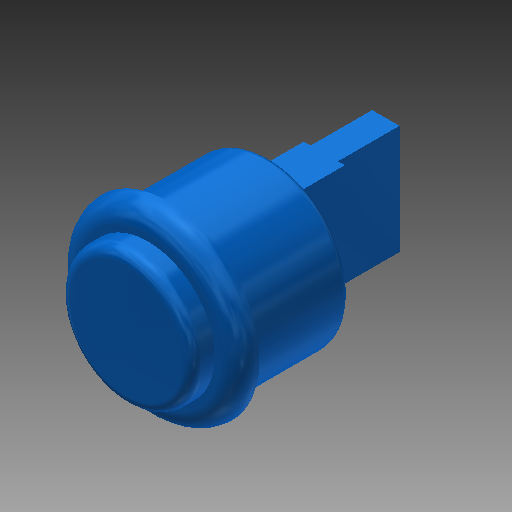
# Autodesk Inventor part: OBSF-24_button
Saved by Autodesk Inventor 2019 (Build 230136000, 136)
## iProperties
Created: 2013-02-11
Part Number: OBSF-24_button
Material: Nylon 6
Document SubType Name: Modeling
Designer: mstine
Density: 1 g/cm^3
Appearance: Nylon 6
Author: mstine
Autodesk Inventor part; units mm, degrees
ref_plane "YZ Plane" through (0, 0, 0) normal (1, 0, 0) x (0, 1, 0)
ref_plane "XZ Plane" through (0, 0, 0) normal (0, 1, 0) x (-1, 0, 0)
ref_plane "XY Plane" through (0, 0, 0) normal (0, 0, 1) x (1, 0, 0)
sketch "Sketch1" plane through (0, 0, 0) normal (0, 0, 1) x (1, 0, 0)
  circle A0 centre (0, 0) radius 11.75
  dimension "d0" = 23.5
  constraints: 1 centre point, 1 coincident
  measures "d0" diameter of A0
extrude "Extrusion1" add sketch "Sketch1" against normal blind 15
sketch "Sketch2" plane through (0, 0, 0) normal (0, 0, 1) x (1, 0, 0)
  circle A0 centre (0, 0) radius 11.75 projected
  circle A1 centre (0, 0) radius 13.5
  dimension "d3" = 27
  constraints: 1 centre point, 1 coincident
  measures "d3" diameter of A1
extrude "Extrusion2" add sketch "Sketch2" along normal blind 2.8 contours A0 | A1
sketch "Sketch3" plane through (0, 0, 2.8) normal (0, 0, 1) x (1, 0, 0)
  circle A0 centre (0, 0) radius 13.5 projected
  circle A1 centre (0, 0) radius 9.75
  dimension "d8" = 19.5
  constraints: 1 centre point, 1 coincident
  measures "d8" diameter of A1
extrude "Extrusion3" add sketch "Sketch3" along normal blind 3.2 contours A1
fillet "Fillet1" radius 1.5 1 edges at (-9.75, 0, 6)
fillet "Fillet2" radius 2.95 1 edges at (-13.5, 0, 2.8)
fillet "Fillet3" radius 1 1 edges at (-11.75, 0, -15)
sketch "Sketch4" plane through (0, 0, -15) normal (0, 0, -1) x (-1, 0, 0)
  circle A0 centre (0, 0) radius 10.75 projected
  line L0 (-3, 8) -> (3, 8)
  line L1 (3, 8) -> (3, -8)
  line L2 (3, -8) -> (-3, -8)
  line L3 (-3, -8) -> (-3, 8)
  point P0 (3, 0)
  point P1 (0, 8)
  dimension "d14" = 6
  dimension "d16" = 16
  constraints: 8 end point, 2 midpoint, 2 parallel, 1 horizontal, 1 horizontal alignment, 1 perpendicular, 1 vertical alignment
  measures "d14" distance of L0.start L0.end
  measures "d16" distance of L0.end L1.end
extrude "Extrusion4" add sketch "Sketch4" along normal blind 8 contours L0 L1 L2 L3
sketch "Sketch5" plane through (0, 0, -23) normal (0, 0, -1) x (-1, 0, 0)
  line L0 (3, 8) -> (-3, 8) projected
  line L1 (3, -8) -> (3, 8) projected
  line L2 (-2, 8) -> (2, 8)
  line L3 (2, 8) -> (2, -8)
  line L4 (2, -8) -> (-2, -8)
  line L5 (-2, -8) -> (-2, 8)
  point P0 (0, 0)
  point P1 (2, 0)
  point P2 (3, 0)
  point P3 (0, 8)
  point P4 (0, 8)
  dimension "d19" = 4
  dimension "d21" = 16
  constraints: 8 end point, 4 midpoint, 2 parallel, 1 coincident, 1 horizontal, 1 horizontal alignment, 1 perpendicular
  measures "d19" distance of L2.start L2.end
  measures "d21" distance of L2.end L3.end
extrude "Extrusion5" add sketch "Sketch5" along normal blind 9
body "Solid1"
